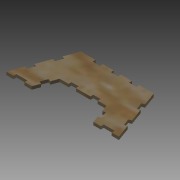
# Autodesk Inventor part: back
Saved by Autodesk Inventor 2015 (Build 190159000, 159)
## iProperties
Created: 2015-10-06
Part Number: back
Material: Generic
Document SubType Name: Modeling
Designer: Haukur
Density: 1 g/cm^3
Appearance: Plywood - Weathered
Author: Haukur
Autodesk Inventor part; units mm, degrees
ref_plane "YZ Plane" through (0, 0, 0) normal (1, 0, 0) x (0, 1, 0)
ref_plane "XZ Plane" through (0, 0, 0) normal (0, 1, 0) x (-1, 0, 0)
ref_plane "XY Plane" through (0, 0, 0) normal (0, 0, 1) x (1, 0, 0)
sketch "Sketch1" plane through (0, 0, 0) normal (0, 0, 1) x (1, 0, 0)
  line L0 (0, 0) -> (80, 0) construction
  line L1 (119.7232, 0) -> (109.4626, 28.1908)
  line L2 (27.3616, 75.1754) -> (20.5212, 56.3816)
  line L3 (20.5212, 56.3816) -> (24.28, 55.0135)
  line L4 (24.28, 55.0135) -> (20.8598, 45.6166)
  line L5 (20.8598, 45.6166) -> (17.101, 46.9846)
  line L6 (17.101, 46.9846) -> (10.2606, 28.1908)
  line L7 (10.2606, 28.1908) -> (14.0194, 26.8227)
  line L8 (14.0194, 26.8227) -> (10.5992, 17.4258)
  line L9 (10.5992, 17.4258) -> (6.8404, 18.7939)
  line L10 (6.8404, 18.7939) -> (0, 0)
  line L11 (27.3616, 75.1754) -> (47.3616, 75.1754)
  line L12 (47.3616, 75.1754) -> (47.3616, 71.1754)
  line L13 (47.3616, 71.1754) -> (57.3616, 71.1754)
  line L14 (57.3616, 71.1754) -> (57.3616, 75.1754)
  line L15 (57.3616, 75.1754) -> (72.3616, 75.1754)
  line L16 (72.3616, 75.1754) -> (72.3616, 71.1754)
  line L17 (72.3616, 71.1754) -> (82.3616, 71.1754)
  line L18 (82.3616, 71.1754) -> (82.3616, 75.1754)
  line L19 (82.3616, 75.1754) -> (97.3616, 75.1754)
  line L20 (97.3616, 75.1754) -> (97.3616, 71.1754)
  line L21 (97.3616, 71.1754) -> (107.3616, 71.1754)
  line L22 (107.3616, 71.1754) -> (107.3616, 75.1754)
  line L23 (107.3616, 75.1754) -> (127.3616, 75.1754)
  line L24 (154.7232, 0) -> (147.8828, 18.7939)
  line L25 (147.8828, 18.7939) -> (144.124, 17.4258)
  line L26 (144.124, 17.4258) -> (140.7038, 26.8227)
  line L27 (140.7038, 26.8227) -> (144.4626, 28.1908)
  line L28 (144.4626, 28.1908) -> (137.6222, 46.9846)
  line L29 (137.6222, 46.9846) -> (133.8634, 45.6166)
  line L30 (133.8634, 45.6166) -> (130.4432, 55.0135)
  line L31 (130.4432, 55.0135) -> (134.202, 56.3816)
  line L32 (134.202, 56.3816) -> (127.3616, 75.1754)
  line L33 (0, 0) -> (10, 0)
  line L34 (10, 0) -> (10, 4)
  line L35 (10, 4) -> (25, 4)
  line L36 (25, 4) -> (25, 0)
  line L37 (35, 0) -> (25, 0)
  line L38 (45.2606, 28.1908) -> (41.8404, 18.7939)
  line L39 (41.8404, 18.7939) -> (38.0816, 20.1619)
  line L40 (38.0816, 20.1619) -> (34.6614, 10.765)
  line L41 (34.6614, 10.765) -> (38.4202, 9.3969)
  line L42 (38.4202, 9.3969) -> (35, 0)
  line L43 (45.2606, 28.1908) -> (57.3616, 28.1908)
  line L44 (57.3616, 28.1908) -> (57.3616, 32.1908)
  line L45 (57.3616, 32.1908) -> (67.3616, 32.1908)
  line L46 (67.3616, 32.1908) -> (67.3616, 28.1908)
  line L47 (109.4626, 28.1908) -> (97.3616, 28.1908)
  line L48 (97.3616, 28.1908) -> (97.3616, 32.1908)
  line L49 (97.3616, 32.1908) -> (87.3616, 32.1908)
  line L50 (87.3616, 32.1908) -> (87.3616, 28.1908)
  line L51 (67.3616, 28.1908) -> (87.3616, 28.1908)
  line L52 (109.4626, 28.1908) -> (112.8828, 18.7939)
  line L53 (112.8828, 18.7939) -> (116.6416, 20.1619)
  line L54 (116.6416, 20.1619) -> (120.0618, 10.765)
  line L55 (120.0618, 10.765) -> (116.303, 9.3969)
  line L56 (116.303, 9.3969) -> (119.7232, 0)
  line L57 (119.7232, 0) -> (129.7232, 0)
  line L58 (129.7232, 0) -> (129.7232, 4)
  line L59 (129.7232, 4) -> (144.7232, 4)
  line L60 (144.7232, 4) -> (144.7232, 0)
  line L61 (154.7232, 0) -> (144.7232, 0)
  dimension "d22" = 80
  dimension "d24" = 100
  dimension "d25" = 80
  dimension "d27" = 35
  dimension "d28" = 30
  dimension "d29" = 35
  dimension "d30" = 30
  dimension "d32" = 20
  dimension "d33" = 4
  dimension "d34" = 10
  dimension "d35" = 20
  dimension "d36" = 10
  dimension "d37" = 20
  dimension "d38" = 4
  dimension "d39" = 10
  dimension "d40" = 15
  dimension "d41" = 10
  dimension "d42" = 15
  dimension "d43" = 10
  dimension "d44" = 20
  dimension "d45" = 4
  dimension "d46" = 10
  dimension "d47" = 20
  dimension "d48" = 10
  dimension "d49" = 10
  dimension "d50" = 4
  dimension "d51" = 15
  dimension "d52" = 10
  dimension "d53" = 4
  dimension "d54" = 10
  dimension "d55" = 12.101
  dimension "d56" = 4
  dimension "d57" = 10
  dimension "d58" = 12.101
  dimension "d59" = 10
  dimension "d60" = 10
  dimension "d62" = 10
  dimension "d63" = 10
  dimension "d64" = 4
  dimension "d65" = 15
  constraints: 124 end point, 22 perpendicular, 9 point on line, 1 collinear, 1 horizontal
  measures "d22" distance of L0.start L2.start
  measures "d24" distance of L2.start L23.end
  measures "d25" distance of L23.end L24.start
  measures "d27" distance of L24.start L1.start
  measures "d28" distance of L1.start L1.end
  measures "d29" distance of L0.start L37.start
  measures "d30" distance of L37.start L38.start
  measures "d32" distance of L2.start L2.end
  measures "d33" distance of L2.end L3.end
  measures "d34" distance of L3.end L4.end
  measures "d35" distance of L5.end L6.end
  measures "d36" distance of L7.end L8.end
  measures "d37" distance of L2.start L11.end
  measures "d38" distance of L11.end L12.end
  measures "d39" distance of L12.end L13.end
  measures "d40" distance of L14.end L15.end
  measures "d41" distance of L16.end L17.end
  measures "d42" distance of L18.end L19.end
  measures "d43" distance of L20.end L21.end
  measures "d44" distance of L24.start L24.end
  measures "d45" distance of L24.end L25.end
  measures "d46" distance of L25.end L26.end
  measures "d47" distance of L27.end L28.end
  measures "d48" distance of L29.end L30.end
  measures "d49" distance of L0.start L33.end
  measures "d50" distance of L33.end L34.end
  measures "d51" distance of L34.end L35.end
  measures "d52" distance of L38.start L38.end
  measures "d53" distance of L38.end L39.end
  measures "d54" distance of L39.end L40.end
  measures "d55" distance of L38.start L43.end
  measures "d56" distance of L43.end L44.end
  measures "d57" distance of L44.end L45.end
  measures "d58" distance of L1.end L47.end
  measures "d59" distance of L48.end L49.end
  measures "d60" distance of L1.end L52.end
  measures "d62" distance of L53.end L54.end
  measures "d63" distance of L1.start L57.end
  measures "d64" distance of L57.end L58.end
  measures "d65" distance of L58.end L59.end
extrude "Extrusion1" add sketch "Sketch1" along normal blind 4 contours L1 L55 L54 L53 L47 L48 L49 L50 L51 L46 L45 L44 L43 L38 L39 L40 L41 L42 L37 L36 L35 L34 L33 L10 L9 L8 L7 L6 L5 L4 L3 L2 L11 L12 L13 L14 L15 L16 L17 L18 L19 L20 L21 L22 L23 L32 L31 L30 L29 L28 L27 L26 L25 L24 L61 L60 L59 L58 L57
body "Solid1"
